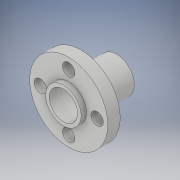
# Autodesk Inventor part: Screw
Saved by Autodesk Inventor 2019 (Build 230136000, 136)
## iProperties
Created: 2019-04-25
Part Number: Screw
Material: Generic
Document SubType Name: Modeling
Designer: 19879326
Density: 1 g/cm^3
Appearance: Default
Author: 19879326
Autodesk Inventor part; units mm, degrees
ref_plane "YZ Plane" through (0, 0, 0) normal (1, 0, 0) x (0, 1, 0)
ref_plane "XZ Plane" through (0, 0, 0) normal (0, 1, 0) x (-1, 0, 0)
ref_plane "XY Plane" through (0, 0, 0) normal (0, 0, 1) x (1, 0, 0)
sketch "Sketch1" plane through (0, 0, 0) normal (1, 0, 0) x (0, 1, 0)
  line L0 (5, 7.5) -> (4, 7.5)
  line L1 (4, 7.5) -> (4, -7.5)
  line L2 (4, -7.5) -> (5, -7.5)
  line L3 (11, 6) -> (5, 6)
  line L4 (5, 2.5) -> (11, 2.5)
  line L5 (11, 2.5) -> (11, 6)
  line L6 (5, -7.5) -> (5, 2.5)
  line L7 (5, 6) -> (5, 7.5)
  line L8 (0, -10.5) -> (0, 10.5) projected
  point P0 (0, 0)
  point P1 (5, 6.75)
  point P2 (5, -2.5)
  point P3 (4, 0)
  dimension "d0" = 10
  dimension "d1" = 3.5
  dimension "d2" = 1.5
  dimension "d3" = 11
  dimension "d4" = 5
  dimension "d5" = 4
  constraints: 16 end point, 4 parallel, 3 midpoint, 2 horizontal, 2 perpendicular, 1 horizontal alignment, 1 vertical alignment
  measures "d0" distance of L2.end L4.start
  measures "d1" distance of L4.end L3.start
  measures "d2" distance of L3.end L0.start
  measures "d3" distance from line of L5 point (0, 0)
  measures "d4" distance from line of L6 point (0, 0)
  measures "d5" distance from line of L1 point (0, 0)
revolve "Revolution1" add sketch "Sketch1" angle 360 about axis through (0, 0, -10) along (0, 0, 1)
sketch "Sketch2" plane through (0, 0, 6) normal (0, 0, 1) x (1, 0, 0)
  circle A0 centre (0, 0) radius 8
  circle A1 centre (0, 8) radius 1.75
  circle A2 centre (8, 0) radius 1.75
  circle A3 centre (-8, 0) radius 1.75
  circle A4 centre (0, -8) radius 1.75
  dimension "d7" = 16
  dimension "d8" = 3.5
  constraints: 5 centre point, 4 point on circle, 3 equal radius, 1 coincident
  measures "d7" diameter of A0
  measures "d8" diameter of A1
extrude "Extrusion1" cut sketch "Sketch2" against normal blind 10 contours A0 A2 | A0 A2 | A1 A0 | A0 A1 | A4 A0 | A0 A4 | A3 A0 | A0 A3
body "Solid1"
